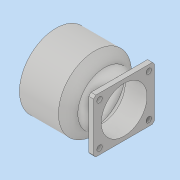
# Autodesk Inventor part: Rohrhalterung_2
Saved by Autodesk Inventor 2018 (Build 220112000, 112)
## iProperties
Created: 2020-05-28
Part Number: Rohrhalterung_2
Material: Generisch
Document SubType Name: Modeling
Designer: marce
Density: 1 g/cm^3
Appearance: Vorgabe
Author: marce
Autodesk Inventor part; units mm, degrees
ref_plane "YZ Plane" through (0, 0, 0) normal (1, 0, 0) x (0, 1, 0)
ref_plane "XZ Plane" through (0, 0, 0) normal (0, 1, 0) x (-1, 0, 0)
ref_plane "XY Plane" through (0, 0, 0) normal (0, 0, 1) x (1, 0, 0)
sketch "Skizze1" plane through (0, 0, 0) normal (0, 0, 1) x (1, 0, 0)
  line L0 (40.05, 37.45) -> (50, 27.5)
  line L1 (50, 27.5) -> (65, 27.5)
  line L2 (65, 27.5) -> (65, 40)
  line L3 (65, 40) -> (70, 40)
  line L4 (70, 40) -> (70, 0)
  line L5 (70, 0) -> (0, 0)
  line L6 (0, 23.5) -> (70, 23.5)
  line L7 (0, 0) -> (0, 37.45)
  line L8 (0, 37.45) -> (40.05, 37.45)
  line L9 (0, 33.45) -> (37.6704, 33.45)
  line L10 (37.6704, 33.45) -> (47.6204, 23.5)
  dimension "d0" = 23.5
  dimension "d2" = 5
  dimension "d3" = 15
  dimension "d6" = 40
  dimension "d7" = 4
  dimension "d34" = 37.45
  dimension "d35" = 135
  dimension "d36" = 70
  dimension "d52" = 4
  constraints: 22 end point, 6 perpendicular, 4 point on line, 2 horizontal, 1 parallel, 1 vertical
  measures "d0" distance between parallel lines of L5 L6
  measures "d2" distance of L2.end L3.end
  measures "d3" distance of L0.end L1.end
  measures "d6" distance between parallel lines of L5 L3
  measures "d7" distance between parallel lines of L6 L1
  measures "d34" distance between parallel lines of L5 L8
  measures "d35" angle of L1 L0
  measures "d36" distance between parallel lines of L4 L7
  measures "d52" distance between parallel lines of L8 L9
revolve "Umdrehung2" add sketch "Skizze1" angle 360 about axis through (70, 0, 0) along (-1, 0, 0) contours L0 L1 L2 L3 L4 L6 L10 L9 L7 L8
sketch "Skizze5" plane through (70, 0, 0) normal (1, 0, 0) x (0, 0, -1)
  circle A0 centre (0, 0) radius 40 projected
  line L0 (-27.5, 29.0474) -> (-27.5, -29.0474)
  line L1 (27.5, 29.0474) -> (27.5, -29.0474)
  line L2 (-24.9687, -31.25) -> (24.9687, -31.25)
  line L3 (-24.9687, 31.25) -> (24.9687, 31.25)
  circle A1 centre (0, 0) radius 37.45 projected
  circle A2 centre (0, 0) radius 40
  point P0 (0, 31.25)
  point P1 (-27.5, 0)
  dimension "d38" = 62.5
  dimension "d40" = 55
  constraints: 8 end point, 4 parallel, 2 midpoint, 1 coincident, 1 horizontal alignment, 1 perpendicular, 1 vertical, 1 vertical alignment, 12 other
  measures "d38" distance between parallel lines of L2 L3
  measures "d40" distance between parallel lines of L1 L0
extrude "Extrusion3" cut sketch "Skizze5" against normal up to surface (5 mm away) contours A0 L1 A1 | L3 A1 A0 | A1 L1 | A0 L2 A1 | L3 A1 | A1 L2 | L0 A1 A0 | L0 A1
sketch "Skizze6" plane through (70, -29.0474, -27.5) normal (1, 0, 0) x (0, 0, -1)
  line L0 (-55, -2.2026) -> (-49, -2.2026)
  line L1 (-49, -2.2026) -> (-49, 3.7974)
  line L2 (-49, 3.7974) -> (-55, 3.7974)
  line L3 (-55, 3.7974) -> (-55, -2.2026)
  line L4 (-55, 60.2974) -> (-49, 60.2974)
  line L5 (-49, 60.2974) -> (-49, 54.2974)
  line L6 (-49, 54.2974) -> (-55, 54.2974)
  line L7 (-55, 54.2974) -> (-55, 60.2974)
  line L8 (0, 60.2974) -> (-6, 60.2974)
  line L9 (-6, 60.2974) -> (-6, 54.2974)
  line L10 (-6, 54.2974) -> (0, 54.2974)
  line L11 (0, 54.2974) -> (0, 60.2974)
  line L12 (0, 3.7974) -> (-6, 3.7974)
  line L13 (-6, 3.7974) -> (-6, -2.2026)
  line L14 (-6, -2.2026) -> (0, -2.2026)
  line L15 (0, -2.2026) -> (0, 3.7974)
  circle A0 centre (-27.5, 29.0474) radius 23.5 projected
  line L16 (0, 0) -> (0, 58.0948) projected
  arc A1 (0, 58.0948) -> (-2.5313, 60.2974) centre (-27.5, 29.0474) ccw projected
  line L17 (-2.5313, 60.2974) -> (-52.4687, 60.2974) projected
  arc A2 (-52.4687, 60.2974) -> (-55, 58.0948) centre (-27.5, 29.0474) ccw projected
  line L18 (-55, 58.0948) -> (-55, 0) projected
  arc A3 (-55, 0) -> (-52.4687, -2.2026) centre (-27.5, 29.0474) ccw projected
  line L19 (-52.4687, -2.2026) -> (-2.5313, -2.2026) projected
  arc A4 (-2.5313, -2.2026) -> (0, 0) centre (-27.5, 29.0474) ccw projected
  line L20 (0, 0) -> (0, 58.0948) projected
  line L21 (-2.5313, 60.2974) -> (-52.4687, 60.2974) projected
  line L22 (-55, 58.0948) -> (-55, 0) projected
  line L23 (-52.4687, -2.2026) -> (-2.5313, -2.2026) projected
  dimension "d43" = 6
  constraints: 32 end point, 8 parallel, 6 collinear, 5 equal length, 4 horizontal, 4 perpendicular, 4 point on line
  measures "d43" distance of L2.end L0.start
hole "Bohrung2" at (70, -25.25, 21.5) at (70, 25.25, 21.5) at (70, 25.25, -21.5) at (70, -25.25, -21.5) direction (-1, 0, 0) diameter 5.5 depth 8 tip angle 118
